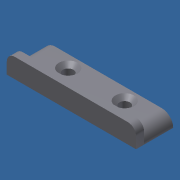
# Autodesk Inventor part: PÁRA-CHOQUE DIANTEIRO
Saved by Autodesk Inventor 2012 SP1 (Build 160190100, 190)
## iProperties
Created: 2012-07-23
Part Number: PÁRA-CHOQUE DIANTEIRO
Material: Carbon Steel
Document SubType Name: Modeling
Designer: bruno.silveira
Density: 7.87 g/cm^3
Mass: 117.106 g
Surface Area: 59.72 cm^2
Volume: 14.88 cm^3
Author: bruno.silveira
Autodesk Inventor part; units mm, degrees
ref_plane "YZ Plane" through (0, 0, 0) normal (1, 0, 0) x (0, 1, 0)
ref_plane "XZ Plane" through (0, 0, 0) normal (0, 1, 0) x (-1, 0, 0)
ref_plane "XY Plane" through (0, 0, 0) normal (0, 0, 1) x (1, 0, 0)
sketch "Sketch1" plane through (0, 0, 0) normal (0, 0, 1) x (1, 0, 0)
  line L0 (0, 0) -> (80, 0)
  line L1 (80, 0) -> (80, 23)
  line L2 (80, 23) -> (0, 23)
  line L3 (0, 23) -> (0, 0)
  dimension "d0" = 80
  dimension "d1" = 23
  constraints: 8 end point, 2 parallel, 1 horizontal, 1 perpendicular
  measures "d0" distance of L1.end L2.end
  measures "d1" distance of L2.end L0.start
extrude "Extrusion1" add sketch "Sketch1" along normal blind 12
sketch "Sketch2" plane through (0, 0, 0) normal (-1, 0, 0) x (0, 0, 1)
  line L0 (0, 23) -> (0, 0) projected
  line L1 (0, 0) -> (12, 0) projected
  line L2 (12, 23) -> (7, 23)
  line L3 (7, 23) -> (7, 5)
  line L4 (7, 5) -> (12, 5)
  line L5 (12, 5) -> (12, 23)
  dimension "d4" = 7
  dimension "d5" = 5
  constraints: 8 end point, 2 parallel, 1 horizontal, 1 perpendicular
  measures "d4" distance between parallel lines of L0 L3
  measures "d5" distance between parallel lines of L1 L4
extrude "Extrusion2" cut sketch "Sketch2" against normal blind 80
sketch "Sketch3" plane through (0, 5, 7) normal (0, 0, 1) x (1, 0, 0)
  line L0 (0, 18) -> (80, 18) projected
  line L1 (0, 0) -> (0, 18) projected
  point P0 (0, -5)
  point P1 (22.5, 10.5)
  point P2 (57.5, 10.5)
  dimension "d8" = 7.5
  dimension "d9" = 7.5
  dimension "d10" = 35
  dimension "d11" = 22.5
  measures "d8" distance from line of L0 point (22.5, 10.5)
  measures "d9" distance from line of L0 point (57.5, 10.5)
  measures "d10" distance of point (22.5, 10.5) point (57.5, 10.5)
  measures "d11" distance from line of L1 point (22.5, 10.5)
hole "Hole1" at (22.5, 15.5, 7) at (57.5, 15.5, 7) direction (0, 0, -1) diameter 6.5 depth 7 tip angle 118 countersink diameter 11.5 countersink angle 90
fillet "Fillet1" radius 7 2 edges at (0, 14, 7) (80, 14, 7)
fillet "Fillet2" radius 5 2 edges at (0, 2.5, 12) (80, 2.5, 12)
body "Solid1"
